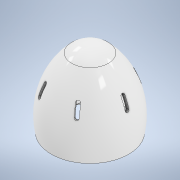
# Autodesk Inventor part: SmartEgg Shell Top
Saved by Autodesk Inventor 2020 (Build 240168000, 168)
## iProperties
Created: 2019-11-26
Part Number: SmartEgg Shell Top
Material: Generic
Document SubType Name: Modeling
Designer: Andrew
Density: 1 g/cm^3
Appearance: White
Author: Andrew
Autodesk Inventor part; units mm, degrees
ref_plane "YZ Plane" through (0, 0, 0) normal (1, 0, 0) x (0, 1, 0)
ref_plane "XZ Plane" through (0, 0, 0) normal (0, 1, 0) x (-1, 0, 0)
ref_plane "XY Plane" through (0, 0, 0) normal (0, 0, 1) x (1, 0, 0)
derived "SmartEgg Shell.ipt"
sketch "Shell Sketch" plane through (0, -10.6204, -14.0095) normal (0, 0.7948428, -0.6068154) x (0, 0.6068154, 0.7948428)
  arc A0 (41.0761, -18.875) -> (29.7061, 33.6321) centre (-5.8251, -1.5465) ccw
  arc A1 (17.6255, -35.2107) -> (30.1255, -31.8614) centre (17.6255, -10.2107) ccw construction
  line L0 (17.6255, -35.2107) -> (17.6255, -31.8614) construction
  line L1 (17.6255, 9) -> (37.2511, 9)
  line L2 (17.6255, 26.5) -> (17.6255, -26.5) construction
  line L3 (35.2511, -26.5) -> (35.9855, -27.1787) construction
  arc A2 (29.7061, 33.6321) -> (17.6255, 38.6714) centre (17.6255, 21.6714) ccw
  line L4 (17.6255, 38.6714) -> (17.6255, 35.8135)
  line L5 (17.6255, 35.8135) -> (22.6255, 35.8135)
  arc A3 (28.2849, 32.225) -> (22.6255, 35.8135) centre (17.6255, 21.6714) ccw
  arc A4 (39.0833, 15.4017) -> (28.2849, 32.225) centre (-5.8251, -1.5465) ccw
  arc A5 (35.2511, 22) -> (30.7511, 26.5) centre (30.7511, 22) ccw construction
  line L6 (37.2511, 9) -> (37.2511, -6.8614)
  line L7 (40.1378, -11.8614) -> (43.0994, -11.8614)
  line L8 (40.2511, 9) -> (40.2511, -11.6114)
  line L9 (40.2511, -11.6114) -> (43.1514, -11.6114)
  line L10 (17.6255, -31.8614) -> (30.1255, -31.8614)
  arc A6 (30.1255, -31.8614) -> (41.0761, -18.875) centre (17.6255, -10.2107) ccw
  line L11 (17.6255, -31.8614) -> (17.6255, 9)
  line L12 (35.2511, -26.5) -> (35.2511, 22) construction
  line L13 (20.9175, 10) -> (17.58, 10) construction
  arc A7 (40.2511, 9) -> (39.0833, 15.4017) centre (22.1205, 9) ccw
  arc A8 (39.2001, -18.1818) -> (40.5683, -13.8614) centre (-5.8251, -1.5465) ccw
  arc A9 (37.2511, -22.204) -> (39.2001, -18.1818) centre (17.6255, -10.2107) ccw
  line L14 (40.5683, -13.8614) -> (37.2511, -13.8614)
  line L15 (37.2511, -13.8614) -> (37.2511, -22.204)
  line L16 (40.1378, -11.8614) -> (37.2511, -6.8614)
  point P0 (17.58, 0)
  point P1 (40.2511, 11.9068)
  point P2 (37.2511, -11.8614)
  point P3 (44.151, 0)
sketch "Thread Sketch" plane through (0, -10.6204, -14.0095) normal (0, 0.7948428, -0.6068154) x (0, 0.6068154, 0.7948428)
  line L0 (37.2511, 9) -> (37.2511, -11.8614) construction
  line L1 (40.2511, 9) -> (40.2511, -11.6114) construction
  line L2 (37.2511, 9) -> (39.7511, 6.5)
  line L3 (39.7511, 6.5) -> (39.7511, 4.5)
  line L4 (39.7511, 4.5) -> (37.2511, 2)
  line L5 (37.2511, 2) -> (37.2511, 9)
  line L6 (40.2511, 4.2929) -> (37.7511, 1.7929)
  line L7 (37.7511, 1.7929) -> (37.7511, -0.2071)
  line L8 (37.7511, -0.2071) -> (40.2511, -2.7071)
  line L9 (40.2511, -2.7071) -> (40.2511, 4.2929)
  line L10 (39.7511, 5.5) -> (37.2511, 5.5) construction
  line L11 (37.7511, 0.7929) -> (40.2511, 0.7929) construction
  point P0 (17.58, 0)
sketch "Thread Mask" plane through (0, -10.6204, -14.0095) normal (0, 0.7948428, -0.6068154) x (0, 0.6068154, 0.7948428)
  line L0 (40.2511, 6.5) -> (37.2511, 6.5)
  line L1 (37.2511, 6.5) -> (37.2511, -11.8614)
  line L2 (37.2511, -11.8614) -> (40.2511, -11.8614)
  line L3 (40.2511, -11.8614) -> (40.2511, 6.5)
  line L4 (37.2511, 9) -> (37.2511, -11.8614) construction
  line L5 (40.2511, 9) -> (40.2511, -11.6114) construction
  point P0 (17.58, 0)
ref_plane "Vent Plane" through (16.5, 14.1404, 18.4237) normal (-0.3609294, -0.5659119, -0.7412649) x (0.8431188, -0.5377274, 0)
sketch "Vent Lookup" plane through (0, -10.6204, -14.0095) normal (0, 0.7948428, -0.6068154) x (0, 0.6068154, 0.7948428)
  arc A0 (41.0761, -18.875) -> (29.7061, 33.6321) centre (-5.8251, -1.5465) ccw
  line L0 (40.8046, 16.5) -> (17.6255, 7.5293)
  line L1 (17.6255, 26.5) -> (17.6255, -26.5) construction
  line L2 (20.9175, 10) -> (17.58, 10) construction
  point P0 (17.58, 0)
revolve "Revolution1" add sketch "Shell Sketch" angle 360 about axis through (-31.8614, 0.075, 0) along (1, 0, 0) contours L9 L8 A7 A4 A3 L5 L4 A2 A0
coil "Coil1" sketch "Thread Sketch" operation add axis through (-31.8614, 0.075, 0) along (-1, 0, 0) pitch 9.4142 turns 3 hand right separate body contours L9 L8 L7 L6
coil "Coil2" sketch "Thread Sketch" operation add axis through (-31.8614, 0.075, 0) along (1, 0, 0) pitch 9.4142 turns 3 hand right bodies 2 contours L9 L8 L7 L6
sketch "Top Thread Mask" plane through (0, -10.6204, -14.0095) normal (0, 0.7948428, -0.6068154) x (0, 0.6068154, 0.7948428)
  arc A0 (40.2511, 9) -> (39.0833, 15.4017) centre (22.1205, 9) ccw projected
  arc A1 (39.0833, 15.4017) -> (28.2849, 32.225) centre (-5.8251, -1.5465) ccw projected
  arc A2 (28.2849, 32.225) -> (22.6255, 35.8135) centre (17.6255, 21.6714) ccw projected
  line L0 (17.6255, 35.8135) -> (22.6255, 35.8135) projected
  line L1 (17.6255, 35.8135) -> (17.6255, -11.6114)
  line L2 (17.6255, -11.6114) -> (40.2511, -11.6114)
  line L3 (40.2511, -11.6114) -> (40.2511, 9)
  line L4 (40.2511, -11.6114) -> (43.1514, -11.6114) construction
  point P0 (17.58, 0)
  constraints: 6 end point, 2 vertical, 1 collinear, 1 perpendicular
revolve "Revolution2" cut sketch "Top Thread Mask" angle 360 about axis through (35.8135, 0.075, 0) along (-1, 0, 0) keep common part bodies 2
sketch "Extra Cutout" plane through (0, -10.6204, -14.0095) normal (0, 0.7948428, -0.6068154) x (0, 0.6068154, 0.7948428)
  line L0 (-5, 9) -> (40.2511, 9) construction
  line L1 (17.6255, 9) -> (43.05, 9)
  line L2 (43.05, 9) -> (43.05, 38.6714)
  line L3 (43.05, 38.6714) -> (17.6255, 38.6714)
  line L4 (17.6255, 38.6714) -> (17.6255, 9)
  arc A0 (41.0761, -18.875) -> (29.7061, 33.6321) centre (-5.8251, -1.5465) ccw construction
  arc A1 (29.7061, 33.6321) -> (17.6255, 38.6714) centre (17.6255, 21.6714) ccw construction
  line L5 (37.2511, -6.3614) -> (37.2511, 0)
  line L6 (37.2511, 0) -> (17.58, 0)
  line L7 (17.58, 0) -> (17.58, -16.6114)
  line L8 (17.58, -16.6114) -> (43.1514, -16.6114)
  line L9 (40.2822, -11.6114) -> (43.1514, -11.6114)
  line L10 (43.1514, -11.6114) -> (43.1514, -16.6114)
  line L11 (40.1378, -11.8614) -> (37.2511, -6.8614) projected
  line L12 (37.2511, -6.3614) -> (40.2822, -11.6114)
  line L13 (40.2511, -11.6114) -> (43.1514, -11.6114) projected
  line L14 (37.2511, 9) -> (37.2511, -6.8614) projected
  dimension "d32" = 5
  dimension "d34" = 0.25
  constraints: 22 end point, 4 perpendicular, 3 parallel, 2 horizontal, 2 vertical, 1 collinear, 1 midpoint, 1 point on circle
  measures "d32" distance of L9.end L8.end
  measures "d34" distance between parallel lines of L11 L12
revolve "Revolution3" cut sketch "Extra Cutout" angle 360 about axis through (38.6714, 0.075, 0) along (-1, 0, 0) bodies 2 contours L4 L3 L2 L1
combine bodies "Combine1" operation type add bodies to combine 1 2
sketch "Sketch6" plane through (16.5, 14.1404, 18.4237) normal (-0.3609294, -0.5659119, -0.7412649) x (0.8431188, -0.5377274, 0)
  line L0 (-3.3902, 1.6028) -> (3.3902, -1.6028) construction
  line L1 (-3.9245, 0.4727) -> (2.856, -2.7329)
  line L2 (3.9245, -0.4727) -> (-2.856, 2.7329)
  arc A0 (-2.856, 2.7329) -> (-3.9245, 0.4727) centre (-3.3902, 1.6028) ccw
  arc A1 (2.856, -2.7329) -> (3.9245, -0.4727) centre (3.3902, -1.6028) ccw
  line L3 (-33.211, 15.7011) -> (1.24, -0.5862) projected
  point P0 (-6.3078, 3.048)
  point P1 (0, 0)
  point P2 (0, 0)
  point P3 (0, 0)
  point P4 (0, 0)
  dimension "d19" = 2.5
  dimension "d20" = 7.5
  constraints: 8 end point, 4 point on circle, 4 tangent, 2 centre point, 1 coincident, 1 collinear, 1 midpoint, 1 parallel
  measures "d19" distance between parallel lines of L2 L1
  measures "d20" distance of L0.start L0.end
extrude "Extrusion1" add sketch "Sketch6" along normal blind 10 separate body
pattern_circular "Circular Pattern1" count 6 over 360 about axis through (-1.5465, 0.075, 0) along (-1, 0, 0) bodies 3
combine bodies "Combine2" operation type subtract main body 1 bodies to subtract 3
revolve "Revolution4" cut sketch "Extra Cutout" angle 360 about axis through (0, 0.0474, -0.0362) along (-1, 0, 0) bodies 1 contours L12 L9 L10 L8 L7 L6 L5
ref_plane "Work Plane2" through (0, -10.6204, -14.0095) normal (0, 0.7948428, -0.6068154) x (0, 0.6068154, 0.7948428)
equation "\"d2\" = 2 * Thread_Pitch"
equation "\"d10\" = 2 * Thread_Pitch"
equation "\"Thread_Pitch\" = 4.707107"
body "Solid1"
